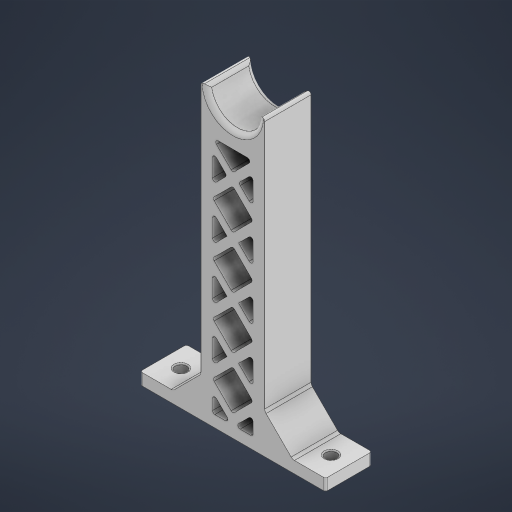
# Autodesk Inventor part: intake_support
Saved by Autodesk Inventor 2024.2 (Build 282272000, 272)
## iProperties
Created: 2025-07-26
Part Number: intake_support
Material: Generic
Document SubType Name: Modeling
Designer: Moe
Density: 1 g/cm^3
Appearance: Default
Author: Moe
Autodesk Inventor part; units mm, degrees
ref_plane "YZ Plane" through (0, 0, 0) normal (1, 0, 0) x (0, 1, 0)
ref_plane "XZ Plane" through (0, 0, 0) normal (0, 1, 0) x (-1, 0, 0)
ref_plane "XY Plane" through (0, 0, 0) normal (0, 0, 1) x (1, 0, 0)
sketch "Sketch1" plane through (0, 0, 0) normal (0, 0, 1) x (1, 0, 0)
  line L0 (0, 0) -> (0, 115)
  circle A0 centre (0, 126.25) radius 11.25
  circle A1 centre (0, 126.25) radius 13.75
  line L1 (-13.75, 126.25) -> (13.75, 126.25)
  line L2 (13.75, 126.25) -> (13.75, 0)
  line L3 (13.75, 0) -> (-13.75, 0)
  line L4 (-13.75, 0) -> (-13.75, 126.25)
  line L5 (0, 0) -> (-40, 0)
  line L6 (-40, 0) -> (-40, 5)
  line L7 (-40, 5) -> (0, 5)
  line L8 (0, 5) -> (0, 0)
  line L9 (0, 5) -> (40, 5)
  line L10 (40, 5) -> (40, 0)
  line L11 (40, 0) -> (0, 0)
  line L12 (0, 0) -> (0, 5)
  point P0 (13.75, 5)
  point P1 (11.25, 126.25)
  point P2 (-11.25, 126.25)
  point P3 (-13.75, 5)
  dimension "d3" = 27.5
  dimension "d0" = 115
  dimension "d1" = 22.5
  dimension "d2" = 11.25
  dimension "d4" = 40
  dimension "d5" = 40
  dimension "d6" = 5
  constraints: 26 end point, 6 parallel, 3 horizontal, 3 perpendicular, 1 centre point, 1 coincident, 1 horizontal alignment, 1 point on line, 1 vertical, 2 other
  measures "d0" distance of L0.start L0.end
  measures "d1" diameter of A0
  measures "d2" distance of L0.end A0.centre
  measures "d4" distance of L6.end L7.end
  measures "d5" distance of L10.end L11.end
  measures "d6" distance of L9.end L10.end
extrude "Extrusion1" add sketch "Sketch1" along normal blind 20 contours L3 L4 L7 L0 | L0 L9 L2 L3 | L7 L4 A1 L0 | L0 A1 L2 L9 | L2 L9 L10 L11 | L5 L6 L7 L4 | A1 L1 A0 L0 | L0 A0 L1 A1
fillet "Fillet1" radius 2 4 edges at (0, 115, 20) (0, 115, 0) (11.25, 126.25, 10) (-11.25, 126.25, 10)
fillet "Fillet2" radius 1 6 edges at (-13.75, 126.25, 10) (13.75, 126.25, 10) (-40, 2.5, 0) (-40, 2.5, 20) (40, 2.5, 20) (40, 2.5, 0)
chamfer "Chamfer1" distance 12 angle 45 2 edges at (-13.75, 5, 10) (13.75, 5, 10)
sketch "Sketch2" plane through (-39, 0, 0) normal (0, -1, 0) x (1, 0, 0)
  line L0 (64.75, 20) -> (64.75, 0) projected
  line L1 (78, 20) -> (64.75, 20) projected
  arc A0 (79, 19) -> (78, 20) centre (78, 19) ccw projected
  line L2 (79, 1) -> (79, 19) projected
  arc A1 (78, 0) -> (79, 1) centre (78, 1) ccw projected
  line L3 (78, 0) -> (64.75, 0) projected
  line L4 (13.25, 0) -> (13.25, 20) projected
  line L5 (13.25, 0) -> (0, 0) projected
  arc A2 (-1, 1) -> (0, 0) centre (0, 1) ccw projected
  line L6 (-1, 1) -> (-1, 19) projected
  arc A3 (0, 20) -> (-1, 19) centre (0, 19) ccw projected
  line L7 (13.25, 20) -> (0, 20) projected
  circle A4 centre (71.375, 10) radius 2.5
  circle A5 centre (6.625, 10) radius 2.5
  point P0 (39, 0)
  point P1 (71.375, 0)
  point P2 (79, 10)
  point P3 (-1, 10)
  dimension "d14" = 5
  dimension "d15" = 5
  dimension "d16" = 10
  dimension "d17" = 7.625
  dimension "d18" = 14.25
  dimension "d19" = 7.625
  dimension "d20" = 7.625
  dimension "d21" = 10
  constraints: 3 midpoint, 2 centre point
  measures "d14" diameter of A4
  measures "d15" diameter of A5
  measures "d16" distance of point (71.375, 0) A4.centre
  measures "d17" distance of point (79, 10) A4.centre
  measures "d18" distance between parallel lines of L0 L2
  measures "d19" distance from line of L2 A4.centre
  measures "d20" distance of point (-1, 10) A5.centre
  measures "d21" distance from line of L5 A5.centre
extrude "Extrusion2" cut sketch "Sketch2" against normal blind 20 contours A4 | A5
fillet "Fillet3" radius 0.5 4 edges at (29.875, 0, 10) (-34.875, 0, 10) (-34.875, 5, 10) (29.875, 5, 10)
fillet "Fillet4" radius 2 4 edges at (-13.75, 17, 10) (-25.75, 5, 10) (25.75, 5, 10) (13.75, 17, 10)
sketch "Sketch3" plane through (0, 0, 0) normal (0, 0, -1) x (-1, 0, 0)
  line L0 (-8.75, 108) -> (8.75, 108)
  line L1 (8.75, 108) -> (8.75, 5)
  line L2 (8.75, 5) -> (-8.75, 5)
  line L3 (-8.75, 5) -> (-8.75, 108)
  line L4 (26.5784, 5) -> (39, 5) projected
  arc A0 (-13.2486, 126.0543) -> (13.2486, 126.0543) centre (0, 126.25) ccw projected
  line L5 (-13.75, 17.8284) -> (-13.75, 125.1874) projected
  line L6 (13.75, 125.1874) -> (13.75, 17.8284) projected
  line L7 (0, 108) -> (0, 5)
  line L8 (-8.75, 108) -> (0, 99.25)
  line L9 (-8.75, 108) -> (3.6244, 108) construction
  line L10 (0, 99.25) -> (8.75, 108)
  line L11 (-8.75, 103) -> (0, 94.25)
  line L12 (0, 94.25) -> (8.75, 103)
  line L13 (0, 99.25) -> (-8.75, 90.5)
  line L14 (0, 94.25) -> (-8.75, 85.5)
  line L15 (-8.75, 85.5) -> (0, 76.75)
  line L16 (-8.75, 85.5) -> (3.6244, 85.5) construction
  line L17 (-8.75, 80.5) -> (0, 71.75)
  line L18 (0, 94.25) -> (8.75, 85.5)
  line L19 (0, 99.25) -> (8.75, 90.5)
  line L20 (8.75, 85.5) -> (0, 76.75)
  line L21 (0, 71.75) -> (8.75, 80.5)
  line L22 (0, 76.75) -> (-8.75, 68)
  line L23 (0, 71.75) -> (-8.75, 63)
  line L24 (0, 76.75) -> (8.75, 68)
  line L25 (0, 71.75) -> (8.75, 63)
  line L26 (8.75, 63) -> (0, 54.25)
  line L27 (-8.75, 63) -> (0, 54.25)
  line L28 (-8.75, 58) -> (0, 49.25)
  line L29 (0, 49.25) -> (8.75, 58)
  line L30 (0, 54.25) -> (-8.75, 45.5)
  line L31 (0, 54.25) -> (8.75, 45.5)
  line L32 (0, 49.25) -> (-8.75, 40.5)
  line L33 (0, 49.25) -> (8.75, 40.5)
  line L34 (-8.75, 40.5) -> (0, 31.75)
  line L35 (8.75, 40.5) -> (0, 31.75)
  line L36 (-8.75, 35.5) -> (0, 26.75)
  line L37 (0, 26.75) -> (8.75, 35.5)
  line L38 (0, 31.75) -> (-8.75, 23)
  line L39 (0, 31.75) -> (8.75, 23)
  line L40 (0, 26.75) -> (-8.75, 18)
  line L41 (0, 26.75) -> (8.75, 18)
  line L42 (8.75, 18) -> (0, 9.25)
  line L43 (-8.75, 18) -> (0, 9.25)
  line L44 (-8.75, 13) -> (0, 4.25)
  line L45 (-8.75, 13) -> (3.6244, 13) construction
  line L46 (0, 4.25) -> (8.75, 13)
  point P0 (0, 0)
  point P1 (0, 113)
  point P2 (-0.75, 5)
  point P3 (0.75, 5)
  point P4 (-2.5, 29.25)
  point P5 (2.5, 29.25)
  point P6 (2.5, 51.75)
  point P7 (-2.5, 51.75)
  point P8 (2.5, 74.25)
  point P9 (-2.5, 74.25)
  point P10 (2.5, 96.75)
  point P11 (-2.5, 96.75)
  dimension "d26" = 0
  dimension "d27" = 5
  dimension "d28" = 5
  dimension "d29" = 5
  dimension "d30" = 45
  dimension "d31" = 5
  dimension "d32" = 5
  dimension "d33" = 45
  dimension "d34" = 5
  dimension "d35" = 5
  dimension "d36" = 5
  dimension "d37" = 5
  dimension "d38" = 45
  dimension "d39" = 5
  dimension "d40" = 5
  constraints: 82 end point, 11 perpendicular, 11 point on line, 7 parallel, 5 horizontal, 3 equal length, 2 midpoint, 1 point on circle, 42 other
  measures "d26" distance between parallel lines of L4 L2
  measures "d27" distance from line of point (0, 113) L0
  measures "d30" angle of L8 L9
  measures "d31" distance of L0.start L11.start
  measures "d32" distance of L0.end L12.end
  measures "d33" angle of L15 L16
  measures "d34" distance of L14.end L17.start
  measures "d35" distance of L18.end L21.end
  measures "d36" distance of L23.end L28.start
  measures "d37" distance of L32.end L36.start
  measures "d38" angle of L44 L45
  measures "d39" distance of L40.end L44.start
  measures "d40" distance of L41.end L46.end
extrude "Extrusion3" cut sketch "Sketch3" against normal blind 20 contours L0 L7 L8 | L0 L10 L7 | L11 L13 L3 | L18 L20 L7 | L7 L15 L14 | L12 L1 L19 | L17 L22 L3 | L25 L26 L7 | L7 L27 L23 | L21 L1 L24 | L33 L35 L7 | L7 L34 L32 | L30 L3 L28 | L29 L1 L31 | L41 L42 L7 | L7 L43 L40 | L38 L3 L36 | L37 L1 L39 | L44 L2 L3 | L1 L2 L46
fillet "Fillet5" radius 1 43 edges at (0, 99.25, 10) (-2.5, 96.75, 10) (2.5, 96.75, 10) (0, 94.25, 10) (0, 71.75, 10) (0, 49.25, 10) (0, 26.75, 10) (0, 76.75, 10) (0, 54.25, 10) (0, 31.75, 10) (0, 9.25, 10) (8.75, 23, 10) (8.75, 18, 10) (8.75, 13, 10) (-8.75, 13, 10) (-8.75, 5, 10) (-0.75, 5, 10) (8.75, 5, 10) (0.75, 5, 10) (-8.75, 18, 10) (-8.75, 23, 10) (-8.75, 58, 10) (-8.75, 35.5, 10) (8.75, 35.5, 10) (8.75, 58, 10) (8.75, 80.5, 10) (8.75, 103, 10) (8.75, 63, 10) (8.75, 40.5, 10) (8.75, 85.5, 10) (8.75, 108, 10) (8.75, 90.5, 10) (8.75, 68, 10) (8.75, 45.5, 10) (-8.75, 45.5, 10) (-8.75, 68, 10) (-8.75, 90.5, 10) (-8.75, 108, 10) (-8.75, 103, 10) (-8.75, 80.5, 10) (-8.75, 40.5, 10) (-8.75, 63, 10) (-8.75, 85.5, 10)
body "Solid1"
